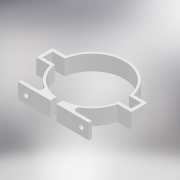
# Autodesk Inventor part: OmegaRing
Saved by Autodesk Inventor 2018.2 (Build 222227000, 227)
## iProperties
Created: 2018-03-27
Part Number: OmegaRing
Material: ABS Plastic
Document SubType Name: Modeling
Designer: mansu
Density: 1.06 g/cm^3
Appearance: Smooth - White
Author: mansu
Autodesk Inventor part; units mm, degrees
ref_plane "YZ Plane" through (0, 0, 0) normal (1, 0, 0) x (0, 1, 0)
ref_plane "XZ Plane" through (0, 0, 0) normal (0, 1, 0) x (-1, 0, 0)
ref_plane "XY Plane" through (0, 0, 0) normal (0, 0, 1) x (1, 0, 0)
sketch "Sketch1" plane through (0, 0, 0) normal (0, 0, 1) x (1, 0, 0)
  circle A0 centre (0, 0) radius 21.15 construction
  line L0 (-18, -25) -> (18, -25) construction
  line L1 (-18, -25) -> (-18, -38.1522) construction
  line L2 (18, -25) -> (18, -38.1522) construction
  line L3 (-23, -23) -> (-23, -25)
  line L4 (-23, -25) -> (-2, -25)
  line L5 (-2, -21.0552) -> (-2, -25)
  line L6 (2, -21.0552) -> (2, -25)
  line L7 (2, -25) -> (23, -25)
  line L8 (23, -25) -> (23, -23)
  line L9 (23, -23) -> (12.7162, -23)
  line L10 (-23, -23) -> (-12.7162, -23)
  arc A1 (2, -21.0552) -> (-2, -21.0552) centre (0, 0) ccw
  arc A2 (11.6803, -19.2892) -> (12.7162, -23) centre (12.7162, -21) ccw
  arc A3 (-12.7162, -23) -> (-11.6803, -19.2892) centre (-12.7162, -21) ccw
  arc A4 (-21.9303, -5.25) -> (-11.6803, -19.2892) centre (0, 0) ccw
  arc A5 (11.6803, -19.2892) -> (21.9303, -5.25) centre (0, 0) ccw
  arc A6 (21.9303, 5.25) -> (-21.9303, 5.25) centre (0, 0) ccw
  line L11 (20.8988, 3.25) -> (28.8988, 3.25)
  line L12 (28.8988, 3.25) -> (28.8988, -3.25)
  line L13 (28.8988, -3.25) -> (20.8988, -3.25)
  line L14 (20.8988, -5.25) -> (30.8988, -5.25)
  line L15 (30.8988, -5.25) -> (30.8988, 5.25)
  line L16 (30.8988, 5.25) -> (20.8988, 5.25)
  line L17 (-21.9303, 5.25) -> (-30.8988, 5.25)
  line L18 (-30.8988, 5.25) -> (-30.8988, -5.25)
  line L19 (-30.8988, -5.25) -> (-21.9303, -5.25)
  line L20 (-20.8988, -3.25) -> (-28.8988, -3.25)
  line L21 (-28.8988, -3.25) -> (-28.8988, 3.25)
  line L22 (-28.8988, 3.25) -> (-20.8988, 3.25)
  point P0 (0, -25)
  point P1 (28.8988, 0)
  point P2 (-28.8988, 0)
  dimension "d13" = 42.3
  dimension "d1" = 25
  dimension "d2" = 36
  dimension "d3" = 2
  dimension "d5" = 5
  dimension "d6" = 2
  dimension "d7" = 4
  dimension "d19" = 22.55
  dimension "d20" = 8
  dimension "d21" = 6.5
  dimension "d22" = 2
  dimension "d23" = 6.5
  dimension "d24" = 8
  dimension "d25" = 2
  dimension "d26" = 2
  dimension "d27" = 2
  constraints: 46 end point, 16 point on circle, 11 perpendicular, 6 centre point, 6 horizontal, 6 point on line, 4 horizontal alignment, 4 tangent, 3 equal radius, 3 midpoint, 2 coincident, 2 vertical, 1 collinear, 1 vertical alignment, 6 other
  measures "d1" distance from line of point (0, 0) L0
  measures "d2" distance of L0.start L0.end
  measures "d3" distance of L7.end L8.end
  measures "d5" distance between parallel lines of L1 L3
  measures "d6" radius of A2
  measures "d7" distance between parallel lines of L5 L6
  measures "d19" radius of A6
  measures "d20" distance of L11.start L11.end
  measures "d21" distance of L11.end L12.end
  measures "d22" distance between parallel lines of L13 L14
  measures "d23" distance of L20.end L21.end
  measures "d24" distance of L21.end L22.end
  measures "d25" distance between parallel lines of L17 L22
  measures "d26" distance between parallel lines of L20 L19
  measures "d27" distance between parallel lines of L18 L21
extrude "Extrusion1" add sketch "Sketch1" along normal blind 10 contours L10 A3 A4 L19 L18 L17 A6 L16 L15 L14 A5 A2 L9 L8 L7 L6 A1 L13 L12 L11 L22 L21 L20 L5 L4 L3
sketch "Sketch2" plane through (2, -25, 0) normal (0, -1, 0) x (1, 0, 0)
  circle A0 centre (16, 5) radius 1.5
  line L0 (21, 0) -> (21, 10) projected
  point P0 (-2, 0)
  point P1 (16, 0)
  point P2 (16, 0)
  point P3 (16, 0)
  point P4 (21, 5)
  dimension "d10" = 3
  constraints: 1 centre point, 1 horizontal alignment, 1 midpoint, 1 vertical alignment
  measures "d10" diameter of A0
extrude "Extrusion2" cut sketch "Sketch2" against normal up to surface (2 mm away)
mirror "Mirror1" about plane through (0, 0, 0) normal (1, 0, 0) of "Extrusion2"
body "Solid1"
